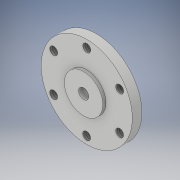
# Autodesk Inventor part: nexus adapter plate final
Saved by Autodesk Inventor 2017 (Build 210142000, 142)
## iProperties
Created: 2017-09-06
Part Number: nexus adapter plate final
Material: Generic
Document SubType Name: Modeling
Designer: User
Density: 1 g/cm^3
Appearance: Default
Author: User
Autodesk Inventor part; units mm, degrees
ref_plane "YZ Plane" through (0, 0, 0) normal (1, 0, 0) x (0, 1, 0)
ref_plane "XZ Plane" through (0, 0, 0) normal (0, 1, 0) x (-1, 0, 0)
ref_plane "XY Plane" through (0, 0, 0) normal (0, 0, 1) x (1, 0, 0)
sketch "Sketch1" plane through (0, 0, 0) normal (0, 0, 1) x (1, 0, 0)
  circle A0 centre (0, 0) radius 28.3972
  dimension "d0" = 56.7944
  constraints: 1 centre point, 1 coincident
  measures "d0" diameter of A0
extrude "Extrusion1" add sketch "Sketch1" along normal blind 5.9944
sketch "Sketch2" plane through (0, 0, 5.9944) normal (0, 0, 1) x (1, 0, 0)
  circle A0 centre (0, 0) radius 11.9888
  dimension "d3" = 23.9776
  constraints: 1 centre point, 1 coincident
  measures "d3" diameter of A0
extrude "Extrusion2" add sketch "Sketch2" along normal blind 1.905
sketch "Sketch3" plane through (0, 0, 7.8994) normal (0, 0, 1) x (1, 0, 0)
  circle A0 centre (0, 0) radius 3.175
  dimension "d6" = 6.35
  constraints: 1 centre point, 1 coincident
  measures "d6" diameter of A0
extrude "Extrusion3" cut sketch "Sketch3" against normal blind 25.4
sketch "Sketch4" plane through (0, 0, 5.9944) normal (0, 0, 1) x (1, 0, 0)
  circle A0 centre (0, 0) radius 28.3972 projected
  circle A1 centre (0, 0) radius 11.9888 projected
  circle A2 centre (0, 0) radius 28.3972 projected
  circle A3 centre (0, 0) radius 28.3972 projected
  point P0 (0.0446, 23.749)
hole "Hole1" at (0.0446, 23.749, 5.9944) direction (0, 0, -1) diameter 4.9784 depth 19.05 tip angle 118 thread size "1/4-20 UNC" class "2B" standard "ANSI Unified Screw Threads"
pattern_circular "Circular Pattern1" count 6 over 360 about axis through (0, 0, 7.8994) along (0, 0, -1) of "Hole1"
body "Solid1"
